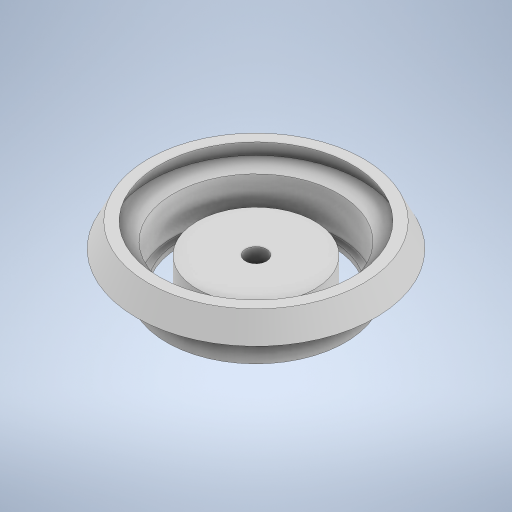
# Autodesk Inventor part: Scroll_nuevo
Saved by Autodesk Inventor 2024.3 (Build 283343000, 343)
## iProperties
Created: 2025-07-29
Part Number: Scroll_nuevo
Material: Genérico
Document SubType Name: Modeling
Designer: eliez
Density: 1 g/cm^3
Appearance: Valor por defecto
Author: eliez
Autodesk Inventor part; units mm, degrees
ref_plane "YZ Plane" through (0, 0, 0) normal (1, 0, 0) x (0, 1, 0)
ref_plane "XZ Plane" through (0, 0, 0) normal (0, 1, 0) x (-1, 0, 0)
ref_plane "XY Plane" through (0, 0, 0) normal (0, 0, 1) x (1, 0, 0)
sketch "Boceto1" plane through (0, 0, 0) normal (0, 1, 0) x (-1, 0, 0)
  circle A0 centre (0, 0) radius 27.5
  dimension "d0" = 55
  constraints: 1 centre point, 1 coincident
  measures "d0" diameter of A0
extrude "Extrusión1" add sketch "Boceto1" along normal blind 10.021
sketch "Boceto2" plane through (0, 10.021, 0) normal (0, 1, 0) x (1, 0, 0)
  circle A0 centre (0, 0) radius 25.5
  dimension "d3" = 51
  constraints: 1 centre point, 1 coincident
  measures "d3" diameter of A0
extrude "Extrusión2" cut sketch "Boceto2" against normal blind 8.447
sketch "Boceto3" plane through (0, 1.574, 0) normal (0, 1, 0) x (1, 0, 0)
  circle A0 centre (0, 0) radius 18.0965
  dimension "d6" = 36.193
  constraints: 1 centre point, 1 coincident
  measures "d6" diameter of A0
extrude "Extrusión3" add sketch "Boceto3" along normal blind 8
sketch "Boceto6" plane through (0, 0, 0) normal (0, -1, 0) x (1, 0, 0)
  circle A0 centre (0, 0) radius 3.25
  dimension "d16" = 6.5
  constraints: 1 centre point, 1 coincident
  measures "d16" diameter of A0
extrude "Extrusión6" cut sketch "Boceto6" against normal blind 10
sketch "Boceto7" plane through (0, 0, 0) normal (0, -1, 0) x (1, 0, 0)
  circle A0 centre (0, 0) radius 3.25 projected
  circle A1 centre (0, 0) radius 10.0335
  dimension "d19" = 20.067
  constraints: 1 centre point, 1 coincident
  measures "d19" diameter of A1
extrude "Extrusión7" cut sketch "Boceto7" against normal blind 4.575
sketch "Boceto10" plane through (0, 0, 0) normal (1, 0, 0) x (0, 1, 0)
  line L0 (10.021, -27.5) -> (10.021, 27.5) projected
  line L1 (10.021, 27.5) -> (11.2756, 27.5)
  line L2 (11.2756, 27.5) -> (11.2756, 36.7936)
  line L3 (11.2756, 36.7936) -> (18.7019, 33.1715)
  line L4 (17.4376, 30.4503) -> (13.2352, 32.5)
  line L5 (10.021, 25.5) -> (1.574, 25.5) projected
  line L6 (10.021, 25.5) -> (13.2352, 25.5)
  line L7 (13.2352, 25.5) -> (13.2352, 32.5)
  line L8 (10.021, 27.5) -> (10.021, 25.5)
  line L9 (26.1838, 0) -> (-2.8727, 0)
  line L10 (17.4376, 30.4503) -> (18.7019, 29.8337)
  line L11 (18.7019, 29.8337) -> (18.7019, 33.1715)
  point P0 (0, 0)
  point P1 (20.2808, 32.4015)
  dimension "d29" = 64
  dimension "d30" = 3
  dimension "d32" = 7
  constraints: 20 end point, 3 perpendicular, 3 point on line, 2 horizontal, 1 collinear, 1 parallel, 1 vertical
  measures "d29" angle of L4 L7
  measures "d30" distance between parallel lines of L3 L4
  measures "d32" distance of L6.end L4.end
revolve "Revolución1" add sketch "Boceto10" angle 360 about axis through (0, 26.1838, 0) along (0, -1, 0)
sketch "Boceto11" plane through (0, 1.574, 0) normal (0, 1, 0) x (1, 0, 0)
  arc A0 (13.0781, 12.5078) -> (13.0781, -12.5078) centre (0, 0) ccw
  arc A1 (17.0129, 16.271) -> (17.0129, -16.271) centre (0, 0) ccw
  arc A2 (17.0129, -16.271) -> (13.0781, -12.5078) centre (15.0455, -14.3894) ccw
  circle A3 centre (0, 0) radius 18.0965 projected
  arc A4 (13.0781, 12.5078) -> (17.0129, 16.271) centre (15.0455, 14.3894) ccw
  constraints: 10 point on circle, 4 centre point, 2 coincident, 2 tangent
extrude "Extrusión10" cut sketch "Boceto11" against normal blind 3 contours A0 A2 A1 A4
